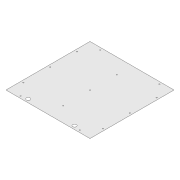
# Autodesk Inventor part: Rückplatte
Saved by Autodesk Inventor 2021.3 (Build 253353000, 353)
## iProperties
Part Number: Rückplatte
Material: PA 6.6
Document SubType Name: Modeling
Designer: SRORF
Mass: 232.891 g
Surface Area: 4108.11 cm^2
Volume: 204.29 cm^3
Density: 1.14 g/cm^3
Appearance: Textur - grau(3)
ROT_Density: 1.0
PDB_Ident_Ver: =<PDB_Ident> <PDB_Version>
ROT_Weight: 0.233 kg
ROT_Weight_Num: 0.23289114062210067
Author: SRORF
Autodesk Inventor part; units mm, degrees
ref_plane "YZ Plane" through (0, 0, 0) normal (1, 0, 0) x (0, 1, 0)
ref_plane "XZ Plane" through (0, 0, 0) normal (0, 1, 0) x (-1, 0, 0)
ref_plane "XY Plane" through (0, 0, 0) normal (0, 0, 1) x (1, 0, 0)
sketch "Skizze2" plane through (0, 0, 0) normal (0, 0, 1) x (1, 0, 0)
  line L0 (-226.5, 226.5) -> (226.5, 226.5)
  line L1 (226.5, 226.5) -> (226.5, -226.5)
  line L2 (226.5, -226.5) -> (-226.5, -226.5)
  line L3 (-226.5, -226.5) -> (-226.5, 226.5)
  point P0 (0, 0)
  point P1 (0, 226.5)
  point P2 (-226.5, 0)
  dimension "d0" = 453
  constraints: 8 end point, 2 midpoint, 2 parallel, 2 perpendicular, 1 horizontal, 1 horizontal alignment, 1 vertical alignment
  measures "d0" distance of L0.start L0.end
extrude "Extrusion1" add sketch "Skizze2" along normal blind 1
sketch "Skizze3" plane through (0, 0, 0) normal (0, 0, -1) x (-1, 0, 0)
  circle A0 centre (125, -208) radius 10
  line L0 (0, -317.1) -> (0, 317.1) projected
  line L1 (226.5, -226.5) -> (-226.5, -226.5) projected
  point P0 (0, 0)
  dimension "d3" = 20
  dimension "d4" = 125
  dimension "d5" = 18.5
  constraints: 1 centre point
  measures "d3" diameter of A0
  measures "d4" distance from line of L0 A0.centre
  measures "d5" distance from line of L1 A0.centre
extrude "Extrusion2" cut sketch "Skizze3" against normal blind 1
pattern_linear "Rechteckige Anordnung1" count 2 spacing 250 along (1, 0, 0) of "Extrusion2"
sketch "Skizze4" plane through (0, 0, 0) normal (0, 0, -1) x (-1, 0, 0)
  point P0 (0, 0)
  point P1 (160, -215)
  point P2 (-160, -215)
  point P3 (-160, 215)
  point P4 (160, 215)
  point P5 (0, 0)
  point P6 (-215, -145)
  point P7 (-215, 0)
  point P8 (-215, 145)
  point P9 (215, 145)
  point P10 (215, 0)
  point P11 (215, -145)
  point P12 (0, 0)
  point P13 (0, -145)
  point P14 (0, 145)
  dimension "d11" = 160
  dimension "d12" = 160
  dimension "d13" = 215
  dimension "d14" = 215
  dimension "d22" = 215
  dimension "d23" = 145
  dimension "d24" = 145
  dimension "d25" = 215
  dimension "d26" = 145
  dimension "d27" = 145
  constraints: 8 vertical alignment, 6 horizontal alignment, 2 coincident
  measures "d11" horizontal distance of point (0, 0) point (160, -215)
  measures "d12" horizontal distance of point (0, 0) point (-160, -215)
  measures "d13" vertical distance of point (0, 0) point (-160, -215)
  measures "d14" vertical distance of point (0, 0) point (-160, 215)
  measures "d22" distance of point (0, 0) point (-215, 0)
  measures "d23" distance of point (-215, 0) point (-215, 145)
  measures "d24" distance of point (-215, 0) point (-215, -145)
  measures "d25" distance of point (0, 0) point (215, 0)
  measures "d26" distance of point (0, 0) point (0, 145)
  measures "d27" distance of point (0, 0) point (0, -145)
hole "Bohrung1" at (0, 0, 0) direction (0, 0, 1) diameter 3.4 depth 15 tip angle 118 countersink diameter 6.3 countersink angle 90 clearance for "Flachkopfsenkschraube" size "M3" standard "Schneeberger VSM"
pattern_sketch "Skizzenbasierte Anordnung1" of "Bohrung1" from (0, 0, 0) copies at (-160, -215, 0) at (160, -215, 0) at (160, 215, 0) at (-160, 215, 0) at (215, -145, 0) at (215, 0, 0) at (215, 145, 0) at (-215, 145, 0) at (-215, 0, 0) at (-215, -145, 0) at (0, -145, 0) at (0, 145, 0)
equation "\"d10\" = 2 * d4"
equation "\"d14\" = d13"
equation "\"d23\" = d24"
equation "\"d25\" = d22"
equation "\"d27\" = d26"
